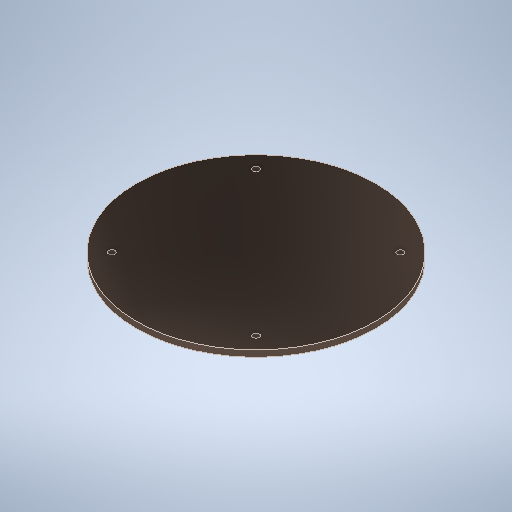
# Autodesk Inventor part: Plataforma
Saved by Autodesk Inventor 2025.2 (Build 292293000, 293)
## iProperties
Created: 2025-11-06
Part Number: Plataforma
Material: Genérico
Document SubType Name: Modeling
Designer: Dax
Density: 1 g/cm^3
Appearance: Gris plomo - Antiguo Pulido
Author: Dax
Autodesk Inventor part; units mm, degrees
ref_plane "YZ Plane" through (0, 0, 0) normal (1, 0, 0) x (0, 1, 0)
ref_plane "XZ Plane" through (0, 0, 0) normal (0, 1, 0) x (-1, 0, 0)
ref_plane "XY Plane" through (0, 0, 0) normal (0, 0, 1) x (1, 0, 0)
sketch "Boceto1" plane through (0, 0, 0) normal (0, 1, 0) x (-1, 0, 0)
  circle A0 centre (0, 0) radius 75
  dimension "d0" = 150
  constraints: 1 centre point, 1 coincident
  measures "d0" diameter of A0
extrude "Extrusión1" add sketch "Boceto1" along normal blind 4
sketch "Boceto2" plane through (0, 4, 0) normal (0, 1, 0) x (1, 0, 0)
  circle A0 centre (0, 0) radius 64
  line L0 (0, 0) -> (64, 0) construction
  circle A1 centre (45.2548, 45.2548) radius 2
  circle A2 centre (-45.2548, 45.2548) radius 2
  circle A3 centre (-45.2548, -45.2548) radius 2
  circle A4 centre (45.2548, -45.2548) radius 2
  dimension "d5" = 4
  dimension "d8" = 360
  constraints: 5 centre point, 2 end point, 1 coincident, 1 horizontal, 9 other
  measures "d5" diameter of A1
extrude "Extrusión2" cut sketch "Boceto2" against normal blind 4 contours A1 A0 | A0 A1 | A4 A0 | A0 A4 | A2 A0 | A0 A2 | A3 A0 | A0 A3
